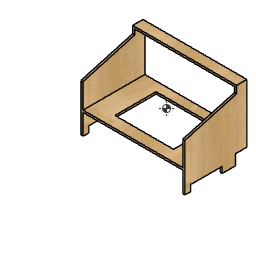
wood_frame (Autodesk Fusion 360 design; units mm, degrees)
Autodesk Fusion 360 part; units mm, degrees
sketch "스케치1" plane through (0, 0, 0) normal (0, 0, 1) x (1, 0, 0)
  line L0 (0, 0) -> (0, 25)
  line L1 (0, 25) -> (50, 25)
  line L2 (50, 25) -> (50, -20)
  line L3 (50, 25) -> (50, -140)
  line L4 (50, -140) -> (50, -20)
  line L5 (50, -140) -> (50, -150)
  line L6 (50, -150) -> (50, -250)
  line L7 (50, -250) -> (-5, -250)
  line L8 (-5, -250) -> (-5, -301)
  line L9 (-5, -301) -> (-70, -301)
  line L10 (-70, -301) -> (-70, -271)
  line L11 (-70, -271) -> (-223, -271)
  line L12 (-223, -271) -> (-223, -301)
  line L13 (-223, -301) -> (-251, -301)
  line L14 (-251, -301) -> (-251, -71)
  line L15 (-251, -71) -> (0, 0)
  dimension "d1" = 25
  dimension "d2" = 50
  dimension "d3" = 45
  dimension "d4" = 165
  dimension "d5" = 120
  dimension "d6" = 10
  dimension "d7" = 100
  dimension "d8" = 55
  dimension "d9" = 51
  dimension "d10" = 65
  dimension "d11" = 30
  dimension "d12" = 153
  dimension "d13" = 30
  dimension "d14" = 28
  dimension "d15" = 230
  constraint coincident L0.start L15.end
  constraint vertical L0
  constraint perpendicular L0 L1
  constraint perpendicular L1 L2
  constraint perpendicular L1 L3
  constraint parallel L3 L4
  constraint parallel L4 L5
  constraint parallel L5 L6
  constraint perpendicular L6 L7
  constraint perpendicular L7 L8
  constraint perpendicular L8 L9
  constraint perpendicular L9 L10
  constraint perpendicular L10 L11
  constraint perpendicular L11 L12
  constraint perpendicular L12 L13
  constraint perpendicular L13 L14
  measures "d1" distance of L0.start L0.end
  measures "d2" distance of L0.end L1.end
  measures "d3" distance of L1.end L2.end
  measures "d4" distance of L1.end L3.end
  measures "d5" distance of L3.end L2.end
  measures "d6" distance of L3.end L5.end
  measures "d7" distance of L5.end L6.end
  measures "d8" distance of L6.end L7.end
  measures "d9" distance of L7.end L8.end
  measures "d10" distance of L8.end L9.end
  measures "d11" distance of L9.end L10.end
  measures "d12" distance of L10.end L11.end
  measures "d13" distance of L11.end L12.end
  measures "d14" distance of L12.end L13.end
  measures "d15" distance of L13.end L14.end
extrude "돌출1" add sketch "스케치1" along normal blind 10 makes body 1
move_body "이동1" bodies 1 to x (0, 1, 0) y (0, 0, 1) z (1, 0, 0) at (-192.0299, 53.7836, 313.2463)
move_body "이동2" bodies 1 to x (1, 0, 0) y (0, 1, 0) z (0, 0, 1) at (0, 0, -11.7)
move_body "이동3" bodies 1 to x (1, 0, 0) y (0, 1, 0) z (0, 0, 1) at (192.0299, 197.2164, -0.5463)
sketch "스케치3" plane through (10, 0, 0) normal (1, 0, 0) x (0, 1, 0)
  line L0 (301, 51) -> (301, 326)
  line L1 (301, 326) -> (251, 326)
  line L2 (251, 326) -> (251, 301)
  line L3 (251, 301) -> (0, 230)
  line L4 (0, 230) -> (0, 0)
  line L5 (0, 0) -> (28, 0)
  line L6 (28, 0) -> (28, 30)
  line L7 (28, 30) -> (181, 30)
  line L8 (181, 30) -> (181, 0)
  line L9 (181, 0) -> (246, 0)
  line L10 (246, 0) -> (246, 51)
  line L11 (246, 51) -> (301, 51)
ref_plane "작업 평면1" through (0, 0, 100) normal (0, 0, 1) x (1, 0, 0)
sketch "스케치4" plane through (0, 0, 100) normal (0, 0, 1) x (1, 0, 0)
  line L0 (0, 0) -> (485, 0)
  line L1 (485, 0) -> (485, 300)
  line L2 (485, 300) -> (0, 300)
  line L3 (0, 300) -> (0, 0)
  line L4 (0, 300) -> (100, 300)
  line L5 (100, 300) -> (100, 255)
  line L6 (0, 0) -> (0, 55)
  line L7 (0, 55) -> (100, 55)
  line L8 (485, 300) -> (385, 300)
  line L9 (385, 300) -> (385, 255)
  line L10 (485, 0) -> (485, 55)
  line L11 (485, 55) -> (385, 55)
  line L12 (100, 255) -> (385, 255)
  line L13 (385, 255) -> (385, 55)
  line L14 (385, 55) -> (100, 55)
  line L15 (100, 55) -> (100, 255)
  dimension "d19" = 485
  dimension "d20" = 300
  dimension "d21" = 100
  dimension "d22" = 45
  dimension "d23" = 55
  dimension "d24" = 100
  dimension "d25" = 100
  dimension "d26" = 45
  dimension "d27" = 55
  dimension "d28" = 100
  constraint horizontal L0
  constraint vertical L1
  constraint horizontal L2
  constraint vertical L3
  constraint coincident L0.start L3.end
  constraint perpendicular L3 L4
  constraint perpendicular L2 L5
  constraint perpendicular L0 L6
  constraint perpendicular L6 L7
  constraint perpendicular L1 L8
  constraint perpendicular L8 L9
  constraint perpendicular L0 L10
  constraint perpendicular L10 L11
  constraint horizontal L12
  constraint vertical L13
  constraint horizontal L14
  constraint vertical L15
  measures "d19" distance of L0.start L0.end
  measures "d20" distance of L0.start L2.end
  measures "d21" distance of L2.end L4.end
  measures "d22" distance of L4.end L5.end
  measures "d23" distance of L0.start L6.end
  measures "d24" distance of L6.end L7.end
  measures "d25" distance of L1.end L8.end
  measures "d26" distance of L8.end L9.end
  measures "d27" distance of L0.end L10.end
  measures "d28" distance of L10.end L11.end
move_body "이동4" bodies 1 to x (1, 0, 0) y (0, 1, 0) z (0, 0, 1) at (-10, 0, 0)
extrude "돌출2" add sketch "스케치4" along normal blind 10 contours L0 L1 L3 L6 L7 L10 L11 L14 | L2 L3 L4 L5 L7 L15 | L1 L2 L8 L9 L11 L13 | L2 L5 L9 L12 bodies 1
split "분할1" by plane through (0, 251, 301) normal (1, 0, 0) bodies 1 makes body 2 at (33.3333, 118.3333, 110)
copy_body "CopyPasteBodies1" bodies 1 makes body 3
move_body "이동5" bodies 3 to x (1, 0, 0) y (0, 1, 0) z (0, 0, 1) at (495, 0, 0)
ref_plane "작업 평면2" through (490, 276, 326) normal (0, 0, 1) x (0, -1, 0)
sketch "스케치5" plane through (0, 0, 326) normal (0, 0, 1) x (1, 0, 0)
  line L0 (0, 0) -> (505, 0)
  line L1 (505, 0) -> (505, 50)
  line L2 (505, 50) -> (0, 50)
  line L3 (0, 50) -> (0, 0)
  dimension "d38" = 505
  dimension "d39" = 50
  constraint horizontal L0
  constraint vertical L1
  constraint horizontal L2
  constraint vertical L3
  constraint coincident L0.start L3.end
  measures "d38" distance of L0.start L0.end
  measures "d39" distance of L0.start L2.end
extrude "돌출3" add sketch "스케치5" along normal blind 10 separate body makes body 4
move_body "이동6" bodies 4 to x (1, 0, 0) y (0, 1, 0) z (0, 0, 1) at (-10, 251, 0)
sketch "스케치6" plane through (0, 0, 110) normal (0, 0, 1) x (-1, 0, 0)
  line L0 (-385, -55) -> (-100, -55)
  line L1 (-100, -55) -> (-100, -255)
  line L2 (-100, -255) -> (-385, -255)
  line L3 (-385, -255) -> (-385, -55)
  line L4 (0, 0) -> (-485, 0)
  line L5 (-485, 0) -> (-485, -300)
  line L6 (-485, -300) -> (0, -300)
  line L7 (0, -300) -> (0, 0)
  line L8 (0, -300) -> (-485, 0)
  line L9 (-485, -300) -> (0, 0)
  line L10 (-242.5, 0) -> (-242.5, -300)
  line L11 (-485, -150) -> (0, -150)
  line L12 (-242.5, -300) -> (0, -150)
  line L13 (-242.5, 0) -> (0, -150)
  line L14 (-242.5, 0) -> (-485, -150)
  line L15 (-242.5, -300) -> (-485, -150)
  line L16 (0, -300) -> (-242.5, 0)
  line L17 (-485, -300) -> (-242.5, 0)
  line L18 (-242.5, -300) -> (0, 0)
  line L19 (-242.5, -300) -> (-485, 0)
  line L20 (-161.6667, -200) -> (-323.3333, -200)
  line L21 (-323.3333, -100) -> (-323.3333, -200)
  line L22 (-323.3333, -100) -> (-161.6667, -100)
  line L23 (-161.6667, -200) -> (-161.6667, -100)
  line L24 (-161.6667, -200) -> (-161.6667, -300)
  line L25 (-323.3333, -200) -> (-323.3333, -300)
  line L26 (-323.3333, -200) -> (-485, -200)
  line L27 (-323.3333, -100) -> (-323.3333, 0)
  line L28 (-323.3333, -100) -> (-485, -100)
  line L29 (-161.6667, -100) -> (0, -100)
  line L30 (-161.6667, -100) -> (-161.6667, 0)
  line L31 (-161.6667, -200) -> (0, -200)
  constraint coincident L6.end L7.start
  constraint coincident L4.end L5.start
  constraint coincident L5.end L6.start
  constraint coincident L4.start L7.end
  constraint midpoint L4 L10.start
  constraint midpoint L6 L10.end
  constraint midpoint L5 L11.start
  constraint midpoint L7 L11.end
  constraint coincident L18 L20.start
  constraint coincident L8 L20.start
  constraint coincident L9 L20.end
  constraint coincident L19 L20.end
  constraint coincident L17 L21.start
  constraint coincident L8 L21.start
  constraint coincident L16 L22.end
  constraint coincident L9 L22.end
  constraint coincident L6 L24.end
  constraint perpendicular L6 L24
  constraint coincident L6 L25.end
  constraint perpendicular L6 L25
  constraint coincident L5 L26.end
  constraint perpendicular L5 L26
  constraint coincident L4 L27.end
  constraint perpendicular L4 L27
  constraint coincident L5 L28.end
  constraint perpendicular L5 L28
  constraint coincident L7 L29.end
  constraint perpendicular L7 L29
  constraint coincident L4 L30.end
  constraint perpendicular L4 L30
  constraint coincident L7 L31.end
  constraint perpendicular L7 L31
move_body "이동7" bodies 1 4 3 to x (1, 0, 0) y (0, 1, 0) z (0, 0, 1) at (0, 350, 0)
pipe "파이프1" add diameter 10 path "스케치6" along L30 separate body makes body 5
pipe "파이프2" add diameter 10 path "스케치6" along L31 separate body makes body 6
pipe "파이프3" add diameter 10 path "스케치6" along L26 separate body makes body 7
pipe "파이프4" add diameter 10 path "스케치6" along L28 separate body makes body 8
pipe "파이프5" add diameter 10 path "스케치6" along L24 bodies 6
pipe "파이프6" add diameter 10 path "스케치6" along L25 bodies 7
pipe "파이프7" add diameter 10 path "스케치6" along L27 bodies 8
pipe "파이프8" add diameter 10 path "스케치6" along L7 L4 L5 L6 bodies 5 6 7 8
pipe "파이프9" add diameter 10 path "스케치6" along L12 bodies 5
pipe "파이프10" add diameter 10 path "스케치6" along L15 bodies 5
pipe "파이프11" add diameter 10 path "스케치6" along L13 bodies 5
pipe "파이프12" add diameter 10 path "스케치6" along L14 bodies 5
pipe "파이프13" add diameter 10 path "스케치6" along L18 bodies 5
pipe "파이프14" add diameter 10 path "스케치6" along L10 bodies 5
pipe "파이프15" add diameter 10 path "스케치6" along L11 bodies 5
pipe "파이프16" add diameter 10 path "스케치6" along L29 bodies 5
pipe "파이프17" add diameter 10 path "스케치6" along L22 bodies 5
pipe "파이프18" add diameter 10 path "스케치6" along L23 bodies 5
pipe "파이프19" add diameter 10 path "스케치6" along L21 bodies 5
pipe "파이프20" add diameter 10 path "스케치6" along L20 bodies 5
pipe "파이프21" add diameter 10 path "스케치6" along L17 bodies 5
pipe "파이프22" add diameter 10 path "스케치6" along L9 bodies 5
pipe "파이프23" add diameter 10 path "스케치6" along L8 bodies 5
pipe "파이프24" add diameter 10 path "스케치6" along L16 bodies 5
pipe "파이프25" add diameter 10 path "스케치6" along L19 bodies 5
move_body "이동8" bodies 5 to x (1, 0, 0) y (0, 1, 0) z (0, 0, 1) at (0, 0, -5)
sketch "스케치7" plane through (0, 0, 336) normal (0, 0, 1) x (-1, 0, 0)
  line L0 (10, -651) -> (10, -601)
  line L1 (10, -601) -> (-495, -601)
  line L2 (-495, -601) -> (-495, -651)
  line L3 (-495, -651) -> (10, -651)
  line L4 (10, -601) -> (-242.5, -651)
  line L5 (-495, -601) -> (-242.5, -651)
  line L6 (-242.5, -601) -> (-242.5, -651)
  constraint coincident L0.end L1.start
  constraint midpoint L3 L4.end
  constraint coincident L1.end L2.start
  constraint midpoint L1 L6.start
pipe "파이프26" add diameter 10 path "스케치7" along L3 separate body makes body 9
pipe "파이프27" add diameter 10 path "스케치7" along L0 L1 L2 L3 bodies 9
pipe "파이프28" add diameter 10 path "스케치7" along L6 bodies 9
pipe "파이프29" add diameter 10 path "스케치7" along L4 bodies 9
pipe "파이프30" add diameter 10 path "스케치7" along L5 bodies 9
move_body "이동9" bodies 9 to x (1, 0, 0) y (0, 1, 0) z (0, 0, 1) at (0, 0, -5)
sketch "스케치8" plane through (495, 0, 0) normal (1, 0, 0) x (0, 1, 0)
  line L0 (350, 230) -> (350, 0)
  line L1 (350, 0) -> (378, 0)
  line L2 (378, 0) -> (378, 30)
  line L3 (378, 30) -> (531, 30)
  line L4 (531, 30) -> (531, 0)
  line L5 (531, 0) -> (596, 0)
  line L6 (596, 0) -> (596, 51)
  line L7 (596, 51) -> (651, 51)
  line L8 (651, 51) -> (651, 326)
  line L9 (651, 326) -> (601, 326)
  line L10 (601, 326) -> (601, 301)
  line L11 (601, 301) -> (350, 230)
  line L12 (651, 230) -> (651, 51)
  line L13 (651, 51) -> (350, 51)
  line L14 (350, 51) -> (350, 230)
  line L15 (350, 230) -> (601, 301)
  constraint vertical L12
  constraint horizontal L13
  constraint vertical L14
  constraint coincident L7.end L8.start
  constraint coincident L0.start L11.end
  constraint parallel L11 L15
move_body "이동10" bodies 5 to x (1, 0, 0) y (0, 1, 0) z (0, 0, 1) at (0, 350, 0)
scale "축척1" factor 0.98 about (242.5, 651, 336) bodies 9
move_body "이동11" bodies 9 to x (1, 0, 0) y (0, 1, 0) z (0, 0, 1) at (0, 0, -5)
delete_body "본체 제거1" bodies 9
delete_body "본체 제거2" bodies 5
move_body "이동12" bodies 2 to x (1, 0, 0) y (0, 1, 0) z (0, 0, 1) at (0, 350, 0)
combine "결합1" operation add target body 1 tool bodies 2 3 4
named bodies: "base_link", "가운데판", "왼판", "우측판", "윗판"
